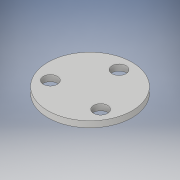
# Autodesk Inventor part: Rotor
Saved by Autodesk Inventor 2018.3 (Build 223284000, 284)
## iProperties
Created: 2018-07-20
Part Number: Rotor
Material: Generisch
Document SubType Name: Modeling
Designer: JochenAlt
Density: 1 g/cm^3
Appearance: Vorgabe
Author: JochenAlt
Autodesk Inventor part; units mm, degrees
ref_plane "YZ Plane" through (0, 0, 0) normal (1, 0, 0) x (0, 1, 0)
ref_plane "XZ Plane" through (0, 0, 0) normal (0, 1, 0) x (-1, 0, 0)
ref_plane "XY Plane" through (0, 0, 0) normal (0, 0, 1) x (1, 0, 0)
sketch "Skizze1" plane through (0, 0, 0) normal (0, 0, 1) x (1, 0, 0)
  line L0 (0, 38.5) -> (0, -38.5) construction
  line L1 (-38.5, 0) -> (38.5, 0) construction
  circle A0 centre (0, 0) radius 19 construction
  circle A1 centre (0, 19) radius 4.6
  circle A2 centre (16.4545, -9.5) radius 4.6
  circle A3 centre (-16.4545, -9.5) radius 4.6
  line L2 (0, 0) -> (-16.4545, -9.5) construction
  line L3 (0, 0) -> (16.4545, -9.5) construction
  circle A4 centre (0, 0) radius 27.5
  dimension "d0" = 9.2
  dimension "d1" = 38
  dimension "d2" = 120
  dimension "d3" = 55
  constraints: 5 centre point, 4 end point, 3 point on circle, 2 coincident, 2 equal radius, 1 point on line, 1 symmetric about line
  measures "d0" diameter of A1
  measures "d1" diameter of A0
  measures "d2" angle of L3 L2
  measures "d3" diameter of A4
extrude "Extrusion1" add sketch "Skizze1" along normal blind 4
